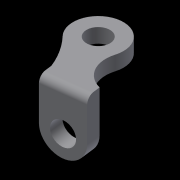
# Autodesk Inventor part: ElbowConnectorUnderlinkLeft
Saved by Autodesk Inventor 2015 (Build 190159000, 159)
## iProperties
Created: 2014-10-15
Part Number: ElbowConnectorUnderlinkLeft
Material: Generic
Document SubType Name: Modeling
Designer: Inventor
Mass: 1.40817 g
Surface Area: 12.256 cm^2
Volume: 1.40817 cm^3
Density: 1 g/cm^3
Appearance: Default
Author: Inventor
Autodesk Inventor part; units mm, degrees
ref_plane "YZ Plane" through (0, 0, 0) normal (1, 0, 0) x (0, 1, 0)
sketch "Base" plane through (0, 0, 0) normal (0, 0, 1) x (1, 0, 0)
  circle A0 centre (0, 0) radius 3.25
  circle A1 centre (0, 0) radius 7
  dimension "d0" = 6.5
  dimension "d1" = 14
  constraints: 2 centre point, 2 coincident
  measures "d0" diameter of A0
  measures "d1" diameter of A1
extrude "BaseFeature" add sketch "Base" along normal blind 4
ref_plane "LinkPlane" through (14.2753, -15.8345, 0) normal (-0.124003, 0.9922818, 0) x (0.9625852, 0.1202919, 0.2428158)
sketch "LinkEnd" plane through (14.2753, -15.8345, 0) normal (-0.124003, 0.9922818, 0) x (0.9625852, 0.1202919, 0.2428158)
  line L0 (-6.4275, 8.6997) -> (-5.2135, 3.8493) construction
  line L1 (-8.3662, 3.0601) -> (-9.5803, 7.9105) construction
  line L2 (-8.3662, 3.0601) -> (-5.2135, 3.8493) construction
  circle A0 centre (-8.9732, 5.4853) radius 3.25
  circle A1 centre (-8.9732, 5.4853) radius 6
  dimension "d21" = 5
  dimension "d23" = 3.25
  dimension "d24" = 5
  dimension "d25" = 6.5
  dimension "d26" = 12
  constraints: 6 end point, 2 centre point, 1 coincident, 1 midpoint, 1 parallel, 1 perpendicular, 2 other
  measures "d21" distance of L1.start L1.end
  measures "d23" distance between parallel lines of L1 L0
  measures "d24" distance from line of L0.start L2
  measures "d25" diameter of A0
  measures "d26" diameter of A1
extrude "LinkEndFeature" add sketch "LinkEnd" along normal blind 4
ref_plane "LowerMountPlane" through (0, 0, 0) normal (0, 0, -1) x (-1, 0, 0)
sketch "LowerMount" plane through (0, 0, 0) normal (0, 0, -1) x (-1, 0, 0)
  line L0 (-9.6884, -12.3766) -> (-3.2385, -13.1827) projected
  line L1 (-0.5098, -13.5237) -> (-12.4171, -12.0356) projected
  circle A0 centre (0, 0) radius 7 projected
  arc A1 (5.0617, -4.8352) -> (-0.5098, -13.5237) centre (24.5854, -23.4853) ccw
  arc A2 (-12.4171, -12.0356) -> (-6.7091, -1.997) centre (-14.3766, -4.2793) ccw
  arc A3 (-6.7091, -1.997) -> (5.0617, -4.8352) centre (0, 0) ccw
  dimension "d27" = 8
  dimension "d28" = 27
  constraints: 8 point on circle, 3 centre point, 3 tangent, 1 concentric
  measures "d27" radius of A2
  measures "d28" radius of A1
extrude "LowerMountFeature" add sketch "LowerMount" against normal up to surface (4 mm away) contours L1 A2 A0 A1 L0
sketch "Link" plane through (6.9595, -16.7488, -7.5) normal (0.124003, -0.9922818, 0) x (0.9922818, 0.124003, 0)
  line L0 (6, 11.5) -> (-6, 11.5) projected
  line L1 (-6, 7.5) -> (-6, 11.5) projected
  line L2 (6, 7.5) -> (-6, 7.5) projected
  line L3 (6, 7.5) -> (6, 11.5) projected
  circle A0 centre (0, 0) radius 6 projected
  line L4 (6, 7.5) -> (6, 0)
  line L5 (-6, 0) -> (-6, 7.5)
  constraints: 4 end point, 2 point on circle, 1 tangent, 1 vertical
extrude "LinkFeature" add sketch "Link" against normal up to surface (4 mm away) contours L3 L2 L1 L0 | L4 A0 L5 L2
fillet "LinkFilletsFeature" radius 2 2 edges at (6.4635, -12.7797, 0) (6.9595, -16.7488, 4)
